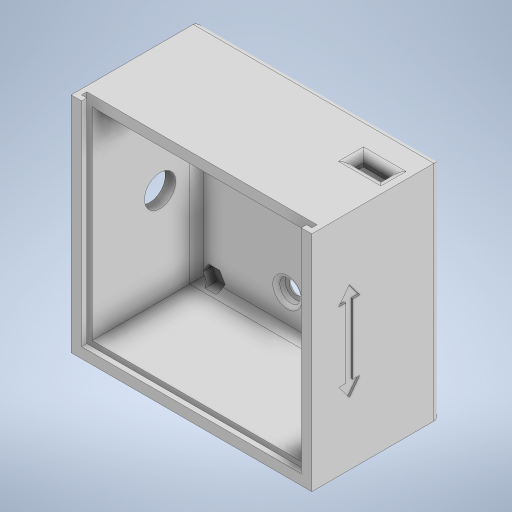
# Autodesk Inventor part: slave
Saved by Autodesk Inventor 2023 (Build 270158000, 158)
## iProperties
Created: 2023-12-06
Part Number: slave
Material: Generic
Document SubType Name: Modeling
Designer: Bruger
Density: 1 g/cm^3
Appearance: Default
Author: Bruger
Autodesk Inventor part; units mm, degrees
ref_plane "YZ Plane" through (0, 0, 0) normal (1, 0, 0) x (0, 1, 0)
ref_plane "XZ Plane" through (0, 0, 0) normal (0, 1, 0) x (-1, 0, 0)
ref_plane "XY Plane" through (0, 0, 0) normal (0, 0, 1) x (1, 0, 0)
sketch "Sketch1" plane through (0, 0, 0) normal (0, 0, 1) x (1, 0, 0)
  line L0 (0, 0) -> (63, 0)
  line L1 (63, 0) -> (63, 58)
  line L2 (63, 58) -> (0, 58)
  line L3 (0, 58) -> (0, 0)
  line L4 (-3, 61) -> (66, 61)
  line L5 (66, 61) -> (66, -3)
  line L6 (66, -3) -> (-3, -3)
  line L7 (-3, -3) -> (-3, 61)
  line L8 (63, 0) -> (58, 0)
  line L9 (26, 54) -> (26, 51.25)
  line L10 (24.4123, 51.25) -> (22.8246, 54)
  line L11 (22.8246, 54) -> (24.4123, 56.75)
  line L12 (24.4123, 56.75) -> (27.5877, 56.75)
  line L13 (27.5877, 56.75) -> (29.1754, 54)
  line L14 (29.1754, 54) -> (27.5877, 51.25)
  line L15 (27.5877, 51.25) -> (24.4123, 51.25)
  line L16 (3.4123, 5.75) -> (1.8246, 3)
  line L17 (1.8246, 3) -> (3.4123, 0.25)
  line L18 (3.4123, 0.25) -> (6.5877, 0.25)
  line L19 (6.5877, 0.25) -> (8.1754, 3)
  line L20 (8.1754, 3) -> (6.5877, 5.75)
  line L21 (6.5877, 5.75) -> (3.4123, 5.75)
  line L22 (53.4123, 5.75) -> (51.8246, 3)
  line L23 (51.8246, 3) -> (53.4123, 0.25)
  line L24 (53.4123, 0.25) -> (56.5877, 0.25)
  line L25 (56.5877, 0.25) -> (58.1754, 3)
  line L26 (58.1754, 3) -> (56.5877, 5.75)
  line L27 (56.5877, 5.75) -> (53.4123, 5.75)
  circle A0 centre (36, 10) radius 5
  circle A1 centre (26, 10) radius 2
  circle A2 centre (26, 10) radius 3.2
  point P0 (5, 0)
  point P1 (5, 3)
  point P2 (55, 3)
  dimension "d0" = 63
  dimension "d1" = 58
  dimension "d2" = 3
  dimension "d3" = 5
  dimension "d9" = 2.75
  constraints: 56 end point, 4 parallel, 3 centre point, 2 coincident, 2 perpendicular, 1 horizontal, 1 midpoint, 1 point on line, 1 vertical, 16 other
  measures "d0" distance of L2.end L1.end
  measures "d1" distance of L1.end L0.end
  measures "d2" distance between parallel lines of L2 L4
  measures "d3" distance of L0.end L8.end
  measures "d9" distance of L9.start L9.end
extrude "Extrusion4" add sketch "Sketch1" along normal blind 35.5 contours L4 L5 L6 L7
extrude "Extrusion5" add sketch "Sketch1" against normal blind 1.5 contours L3 L2 L1 L0 | L4 L5 L6 L7 | L10 L11 L12 L13 L14 L15 | L21 L20 L19 L18 L17 L16 | L27 L26 L25 L24 L23 L22 | A2
extrude "Extrusion6" add sketch "Sketch1" along normal blind 2.5 contours L3 L2 L1 L0
sketch "Sketch3" plane through (-3, 61, 35.5) normal (0, 1, 0) x (1, 0, 0)
  line L0 (69, 37) -> (69, 0) projected
  line L1 (69, 35.5) -> (69, 27)
  line L2 (69, 27) -> (65, 27)
  line L3 (65, 27) -> (65, 23.8)
  line L4 (65, 23.8) -> (56.8, 23.8)
  line L5 (56.8, 23.8) -> (56.8, 27)
  line L6 (56.8, 27) -> (65, 27)
  point P0 (3, 35.5)
  dimension "d29" = 8.5
  dimension "d30" = 4
  dimension "d31" = 3.2
  dimension "d32" = 8.2
  constraints: 12 end point, 4 perpendicular, 3 point on line, 1 collinear
  measures "d29" distance of L1.start L1.end
  measures "d30" distance of L1.end L2.end
  measures "d31" distance of L2.end L3.end
  measures "d32" distance of L3.end L4.end
extrude "Extrusion7" cut sketch "Sketch3" against normal blind 5
fillet "Fillet1" radius 2 4 edges at (57.9, 61, 8.5) (62, 61, 10.1) (57.9, 61, 11.7) (53.8, 61, 10.1)
sketch "Sketch5" plane through (-3, -3, 35.5) normal (-1, 0, 0) x (0, 0, 1)
  line L0 (-37, 64) -> (0, 64) projected
  line L1 (-35.5, 64) -> (-27, 64)
  line L2 (-27, 64) -> (-27, 26)
  line L3 (-33, 61) -> (0, 61) projected
  line L4 (-27, 26) -> (-18, 26)
  line L5 (-18, 26) -> (-18, 35)
  line L6 (-18, 35) -> (-27, 35)
  circle A0 centre (-22.5, 30.5) radius 4.5
  point P0 (-35.5, 3)
  dimension "d36" = 8.5
  dimension "d37" = 38
  dimension "d38" = 90
  dimension "d39" = 9
  dimension "d40" = 9
  constraints: 10 end point, 4 perpendicular, 3 point on line, 1 centre point, 1 tangent
  measures "d36" distance of L1.start L1.end
  measures "d37" distance of L1.end L2.end
  measures "d38" angle of L1 L2
  measures "d39" distance of L2.end L4.end
  measures "d40" distance of L4.end L5.end
extrude "Extrusion8" cut sketch "Sketch5" against normal blind 5 contours A0
sketch "Sketch6" plane through (-3, 61, 35.5) normal (0, 1, 0) x (1, 0, 0)
  line L0 (66, 0) -> (3, 0) projected
  line L1 (66, 33) -> (66, 0) projected
  line L2 (3, 0) -> (66, 0)
  line L3 (66, 0) -> (66, 3)
  line L4 (66, 3) -> (3, 3)
  line L5 (3, 3) -> (3, 0)
  line L6 (66, 3) -> (67.5, 3)
  line L7 (67.5, 3) -> (67.5, 1.5)
  line L8 (67.5, 1.5) -> (66, 1.5)
  line L9 (66, 1.5) -> (66, 3)
  line L10 (3, 3) -> (1.5, 3)
  line L11 (1.5, 3) -> (1.5, 1.5)
  line L12 (1.5, 1.5) -> (3, 1.5)
  line L13 (3, 1.5) -> (3, 3)
  point P0 (3, 35.5)
  point P1 (3, 1.5)
  point P2 (66, 1.5)
  dimension "d43" = 3
  dimension "d44" = 1.5
  dimension "d45" = 1.5
  dimension "d46" = 1.5
  constraints: 24 end point, 6 parallel, 3 horizontal, 3 perpendicular, 2 point on line
  measures "d43" distance of L3.end L2.end
  measures "d44" distance of L7.end L8.end
  measures "d45" distance of L6.end L7.end
  measures "d46" distance of L12.end L11.end
extrude "Extrusion9" cut sketch "Sketch6" against normal up to surface (61 mm away)
sketch "Sketch7" plane through (0, 0, 35.5) normal (0, 1, 0) x (1, 0, 0)
  line L0 (-1.5, 1.5) -> (-1.5, 3) projected
  line L1 (63, 3) -> (64.5, 3) projected
  line L2 (-1.5, 1.5) -> (64.5, 1.5)
  line L3 (64.5, 1.5) -> (64.5, 3)
  line L4 (64.5, 3) -> (-1.5, 3)
  line L5 (-1.5, 3) -> (-1.5, 1.5)
  point P0 (0, 35.5)
  constraints: 8 end point, 2 parallel, 1 horizontal, 1 perpendicular
extrude "Extrusion10" cut sketch "Sketch7" against normal blind 1.5
sketch "Sketch9" plane through (-3, -3, 35.5) normal (-1, 0, 0) x (0, 0, 1)
  line L0 (-9.7363, 32) -> (-11.7363, 32)
  line L1 (-11.7363, 32) -> (-11.7363, 22)
  line L2 (-11.7363, 22) -> (-9.7363, 22)
  line L3 (-9.7363, 22) -> (-9.7363, 32)
  line L4 (-11.7363, 32) -> (-9.7363, 32)
  line L5 (-9.7363, 32) -> (-9.7363, 42)
  line L6 (-9.7363, 42) -> (-11.7363, 42)
  line L7 (-11.7363, 42) -> (-11.7363, 32)
  line L8 (-9.7363, 42) -> (-7.7363, 42)
  line L9 (-7.7363, 42) -> (-10.7363, 46)
  line L10 (-11.7363, 42) -> (-13.7363, 42)
  line L11 (-13.7363, 42) -> (-10.7363, 46)
  line L12 (-9.7363, 22) -> (-7.7363, 22)
  line L13 (-7.7363, 22) -> (-10.7363, 18)
  line L14 (-10.7363, 18) -> (-13.7363, 22)
  line L15 (-13.7363, 22) -> (-11.7363, 22)
  point P0 (-35.5, 3)
  dimension "d51" = 2
  dimension "d52" = 10
  dimension "d53" = 10
  dimension "d54" = 2
  dimension "d55" = 5
  dimension "d56" = 2
  constraints: 32 end point, 7 equal length, 4 horizontal, 3 point on line, 2 perpendicular
  measures "d51" distance of L2.end L1.end
  measures "d52" distance of L1.end L0.end
  measures "d53" distance of L5.end L4.end
  measures "d54" distance of L5.end L8.end
  measures "d55" distance of L8.end L9.end
  measures "d56" distance of L6.end L10.end
extrude "Extrusion11" cut sketch "Sketch9" against normal blind 0.5
sketch "Sketch10" plane through (66, -3, 35.5) normal (1, 0, 0) x (0, 0, -1)
  line L0 (37, 0) -> (0, 0) projected
  line L1 (0, 0) -> (0, 5.4567)
  line L2 (0, 64) -> (0, 0) projected
  line L3 (11.7363, 32) -> (11.7363, 22)
  line L4 (9.7363, 22) -> (9.7363, 32)
  line L5 (9.7363, 32) -> (11.7363, 32)
  line L6 (11.7363, 32) -> (9.7363, 32)
  line L7 (11.7363, 42) -> (11.7363, 32)
  line L8 (9.7363, 32) -> (9.7363, 42)
  line L9 (11.7363, 42) -> (13.7363, 42)
  line L10 (9.7363, 42) -> (11.7363, 42)
  line L11 (9.7363, 42) -> (7.7363, 42)
  line L12 (13.7363, 42) -> (10.7363, 46)
  line L13 (7.7363, 42) -> (10.7363, 46)
  line L14 (11.7363, 22) -> (9.7363, 22)
  line L15 (9.7363, 22) -> (7.7363, 22)
  line L16 (13.7363, 22) -> (11.7363, 22)
  line L17 (7.7363, 22) -> (10.7363, 18)
  line L18 (10.7363, 18) -> (13.7363, 22)
  point P0 (35.5, 3)
  constraints: 34 end point, 4 point on line
extrude "Extrusion12" cut sketch "Sketch10" against normal blind 0.5
sketch "Sketch11" plane through (0, 0, -1.5) normal (0, 0, -1) x (-1, 0, 0)
  line L0 (-56.4588, 39.8242) -> (-6.5412, 39.8242) construction
  line L1 (-6.5412, 39.8242) -> (-6.5412, 18.1758) construction
  line L2 (-6.5412, 18.1758) -> (-56.4588, 18.1758) construction
  line L3 (-56.4588, 18.1758) -> (-56.4588, 39.8242) construction
  line L4 (-66, -3) -> (-66, 61) projected
  line L5 (3, -3) -> (-66, -3) projected
  line L6 (-10.5568, 20.6097) -> (-10.5568, 38.264)
  line L7 (-10.5568, 38.264) -> (-15.8928, 38.264)
  line L8 (-15.8928, 29.4368) -> (-15.8928, 20.6097)
  line L9 (-15.8928, 20.6097) -> (-10.5568, 20.6097)
  line L10 (-10.5568, 20.6097) -> (-10.5568, 38.264)
  line L11 (-25.0304, 20.6097) -> (-25.0304, 29.4368)
  line L12 (-25.0304, 29.4368) -> (-20.6364, 22.7599)
  line L13 (-20.6364, 22.7599) -> (-15.8928, 29.4368)
  line L14 (-20.6364, 30.864) -> (-15.8928, 38.264)
  line L15 (-20.6364, 30.864) -> (-25.0304, 38.264)
  arc A0 (-25.7497, 36.4397) -> (-30.1499, 38.264) centre (-31.245, 29.4038) ccw
  arc A1 (-27.8259, 32.6258) -> (-34.3988, 33.8694) centre (-32.9359, 23.6093) ccw
  arc A2 (-34.3988, 33.8694) -> (-34.3988, 32.0662) centre (-34.0519, 32.9678) ccw
  arc A3 (-26.8336, 29.9106) -> (-34.3988, 32.0662) centre (-34.1757, 18.496) ccw
  arc A4 (-26.9903, 21.5552) -> (-26.8336, 29.9106) centre (-31.0786, 25.8111) ccw
  arc A5 (-29.3483, 20.6097) -> (-26.9903, 21.5552) centre (-30.3156, 26.435) ccw
  line L16 (-25.7497, 36.4397) -> (-27.8259, 32.6258)
  arc A6 (-31.5, 24.7895) -> (-31.5, 26.6338) centre (-31.6052, 25.7116) ccw
  arc A7 (-38.7729, 29) -> (-31.5, 26.6338) centre (-29.6873, 44.5656) ccw
  arc A8 (-40.0752, 30.7187) -> (-38.7729, 29) centre (-37.8861, 31.0247) ccw
  arc A9 (-38.7729, 26.435) -> (-34.1757, 24.7895) centre (-34.2488, 31.8299) ccw
  line L17 (-34.1757, 24.7895) -> (-31.5, 24.7895)
  line L18 (-38.7729, 26.435) -> (-40.7323, 22.5075)
  line L19 (-40.7323, 22.5075) -> (-39.2862, 21.5552)
  arc A10 (-43.6059, 20.2997) -> (-39.2862, 21.5552) centre (-43.7468, 28.8432) ccw
  line L20 (-43.6059, 20.2997) -> (-46.5138, 20.2997)
  arc A11 (-54.3214, 28.3167) -> (-46.5138, 20.2997) centre (-46.3015, 28.3167) ccw
  arc A12 (-45.7045, 38.6087) -> (-54.3214, 30.1885) centre (-45.899, 30.1885) ccw
  line L21 (-45.7045, 38.6087) -> (-44.0209, 38.6087)
  arc A13 (-38.8098, 36.9732) -> (-44.0209, 38.6087) centre (-44.0209, 29.4895) ccw
  arc A14 (-38.8098, 36.9732) -> (-40.3838, 33.408) centre (-35.4044, 33.3398) ccw
  line L22 (-40.3838, 33.408) -> (-40.3838, 31.8299)
  line L23 (-40.3838, 31.8299) -> (-40.7323, 31.5485)
  arc A15 (-40.7323, 31.5485) -> (-43.9249, 33.9854) centre (-44.3814, 30.0775) ccw
  line L24 (-43.9249, 33.9854) -> (-45.6282, 33.9854)
  arc A16 (-45.6282, 33.9854) -> (-48.9095, 30.1885) centre (-45.1447, 30.2512) ccw
  line L25 (-48.9095, 30.1885) -> (-48.9095, 28.3167)
  arc A17 (-48.9095, 28.3167) -> (-45.4646, 24.7895) centre (-45.3716, 28.3262) ccw
  line L26 (-45.4646, 24.7895) -> (-44.0209, 24.7895)
  arc A18 (-44.0209, 24.7895) -> (-41.3619, 27.0474) centre (-44.2569, 27.762) ccw
  line L27 (-41.3619, 27.0474) -> (-45.7045, 27.0474)
  line L28 (-45.7045, 27.0474) -> (-45.7045, 30.7187)
  line L29 (-45.7045, 30.7187) -> (-40.0752, 30.7187)
  line L30 (-25.0304, 20.6097) -> (-29.3483, 20.6097)
  line L31 (-54.3214, 28.3167) -> (-54.3214, 30.1885)
  line L32 (-30.1499, 38.264) -> (-25.0304, 38.264)
  point P0 (0, 0)
  point P1 (-31.5, 29)
  point P2 (-31.5, 29)
  constraints: 54 end point, 40 point on circle, 19 centre point, 8 horizontal, 5 perpendicular, 3 vertical, 2 parallel, 1 point on line, 1 tangent, 2 other
extrude "Extrusion13" cut sketch "Sketch11" against normal blind 0.5
fillet "Fillet2" radius 2 8 edges at (66, 29, -1.5) (31.5, 61, -1.5) (-3, 29, -1.5) (31.5, -3, -1.5) (31.5, 0, 2.5) (0, 29, 2.5) (31.5, 58, 2.5) (63, 29, 2.5)
fillet "Fillet3" radius 2 2 edges at (31, 10, -1.5) (24, 10, -1.5)
fillet "Fillet4" radius 1 2 edges at (31, 10, 2.5) (22.8, 10, 2.5)
body "Solid1"
